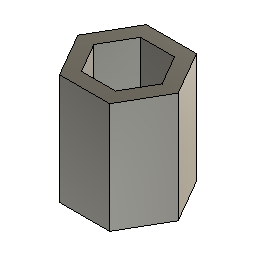
Motor Joint Adapter (Autodesk Fusion 360 design; units mm, degrees)
Autodesk Fusion 360 part; units mm, degrees
sketch "Sketch1" plane through (0, 0, 0) normal (0, 0, 1) x (1, 0, 0)
  line L0 (0, 0) -> (3.4, 0)
  line L1 (3.4, 0) -> (6.8, 5.889)
  line L2 (6.8, 5.889) -> (3.4, 11.7779)
  line L3 (3.4, 11.7779) -> (-3.4, 11.7779)
  line L4 (-3.4, 11.7779) -> (-6.8, 5.889)
  line L5 (-6.8, 5.889) -> (-3.4, 0)
  line L6 (-3.4, 0) -> (3.4, 0)
  point P0 (0, 5.889)
  dimension "d1" = 3.4
  dimension "d2" = 6.8
  constraint coincident L0.start origin
  constraint horizontal L0
  measures "d1" distance of L0.start L0.end
  measures "d2" distance of L0.end L5.end
extrude "Extrude1" add sketch "Sketch1" along normal blind 10
sketch "Sketch2" plane through (0, 0, 10) normal (0, 0, 1) x (-1, 0, 0)
  line L0 (3.4, 0) -> (-3.4, 0)
  line L1 (-3.4, 0) -> (-6.8, -5.889)
  line L2 (-6.8, -5.889) -> (-3.4, -11.7779)
  line L3 (-3.4, -11.7779) -> (3.4, -11.7779)
  line L4 (3.4, -11.7779) -> (6.8, -5.889)
  line L5 (6.8, -5.889) -> (3.4, 0)
  line L6 (-3.4, 0) -> (3.4, -11.7779)
  line L7 (-3.4, 0) -> (0, -5.889)
  line L8 (0, -5.889) -> (-2.05, -2.3383)
  line L9 (-2.05, -2.3383) -> (-4.1, -5.889)
  line L10 (-4.1, -5.889) -> (-2.05, -9.4397)
  line L11 (-2.05, -9.4397) -> (2.05, -9.4397)
  line L12 (2.05, -9.4397) -> (4.1, -5.889)
  line L13 (4.1, -5.889) -> (2.05, -2.3383)
  line L14 (2.05, -2.3383) -> (-2.05, -2.3383)
  line L15 (-2.05, -2.3383) -> (-2.0499, -2.3383) construction
  point P0 (0.025, -5.9323)
  point P1 (0, -5.889)
  dimension "d10" = 6.8
  dimension "d11" = 4.1
  dimension "d12" = 4.1
  dimension "d13" = 0
  constraint coincident L0.end L1.start
  constraint coincident L3.end L4.start
  constraint midpoint L6 P1
  constraint parallel L6 L8
  constraint horizontal L15
  measures "d10" distance of L0.end P1
  measures "d11" distance of P1 L8.end
  measures "d12" distance of L8.end L13.end
  measures "d13" angle of L14 L15
extrude "Extrude2" add sketch "Sketch2" along normal blind 5 contours L6 L7 L8 L12 L13 L14 | L6 L7 L8 L9 L10 L11
extrude "Extrude3" add 1 faces at (-0.6833, 0.7794, 10) along direction (0, 0, 1) blind 6
extrude "Extrude4" cut 1 faces at (0.6833, 4.7054, 15) along direction (0, 0, -1) blind 10
extrude "Extrude5" cut 1 faces at (-0.6833, 0.7794, 16) along direction (0, 0, -1) blind 1
sketch "Sketch3" plane through (0, 0, 5) normal (0, 0, 1) x (-1, 0, 0)
  line L0 (2.05, -2.3383) -> (-2.05, -2.3383)
  line L1 (-2.05, -2.3383) -> (-4.1, -5.889)
  line L2 (-4.1, -5.889) -> (-2.05, -9.4397)
  line L3 (-2.05, -9.4397) -> (2.05, -9.4397)
  line L4 (2.05, -9.4397) -> (4.1, -5.889)
  line L5 (4.1, -5.889) -> (2.05, -2.3383)
  line L6 (-2.05, -9.4397) -> (0, -5.889)
  circle A0 centre (0, -5.889) radius 1.5
  dimension "d22" = 3
  constraint coincident L2.end L3.start
  constraint coincident L6.end A0.centre
  measures "d22" diameter of A0
extrude "Extrude6" cut sketch "Sketch3" against normal blind 5 contours A0
sketch "Sketch4" plane through (0, 0, 15) normal (0, 0, 1) x (-1, 0, 0)
  line L0 (2.05, -2.3383) -> (4.1, -5.889)
  line L1 (4.1, -5.889) -> (2.05, -9.4397)
  line L2 (2.05, -9.4397) -> (-2.05, -9.4397)
  line L3 (-2.05, -9.4397) -> (-4.1, -5.889)
  line L4 (-4.1, -5.889) -> (-2.05, -2.3383)
  line L5 (-2.05, -2.3383) -> (2.05, -2.3383)
  line L6 (3.4, 0) -> (-3.4, 0)
  line L7 (-3.4, 0) -> (-6.8, -5.889)
  line L8 (-6.8, -5.889) -> (-3.4, -11.7779)
  line L9 (-3.4, -11.7779) -> (3.4, -11.7779)
  line L10 (3.4, -11.7779) -> (6.8, -5.889)
  line L11 (6.8, -5.889) -> (3.4, 0)
  line L12 (-2.05, -2.3383) -> (2.05, -9.4397)
  line L13 (2.05, -9.4397) -> (0, -5.889)
  line L14 (-2.05, -2.3383) -> (0, -5.889)
  line L15 (0, -5.889) -> (-2.3125, -1.8836)
  line L16 (-2.3125, -1.8836) -> (-4.625, -5.889)
  line L17 (-4.625, -5.889) -> (-2.3125, -9.8943)
  line L18 (-2.3125, -9.8943) -> (2.3125, -9.8943)
  line L19 (2.3125, -9.8943) -> (4.625, -5.889)
  line L20 (4.625, -5.889) -> (2.3125, -1.8836)
  line L21 (2.3125, -1.8836) -> (-2.3125, -1.8836)
  point P0 (0, -5.889)
  dimension "d25" = 4.625
  dimension "d26" = 4.625
  constraint coincident L4.end L5.start
  constraint coincident L1.end L2.start
  constraint midpoint L12 P0
  constraint parallel L14 L15
  measures "d25" distance of P0 L15.end
  measures "d26" distance of L15.end L20.end
extrude "Extrude7" cut sketch "Sketch4" against normal blind 10 contours L16 L17 L18 L19 L20 L21
extrude "Extrude8" cut 1 faces at (0.0374, 1.4644, 0) along direction (0, 0, 1) blind 2
extrude "Extrude9" add 1 faces at (0.7708, 0.6279, 15) along direction (0, 0, 1) blind 2
